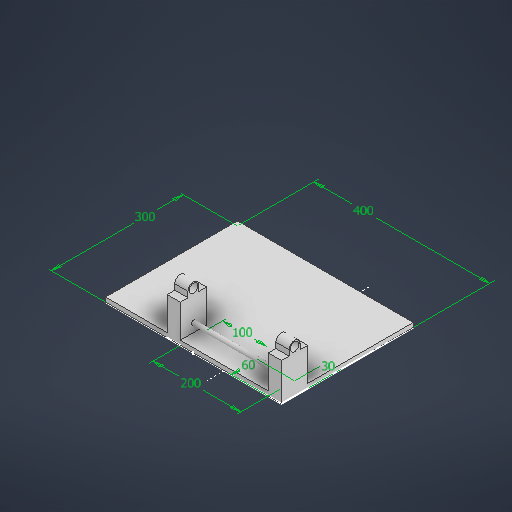
# Autodesk Inventor part: base
Saved by Autodesk Inventor 2026.1 (Build 301233020, 233B)
## iProperties
Created: 2025-12-30
Part Number: base
Material: Generic
Document SubType Name: Modeling
Designer: Austin Ngobeni
Density: 1 g/cm^3
Appearance: Default
Author: Austin Ngobeni
Autodesk Inventor part; units mm, degrees
ref_plane "YZ Plane" through (0, 0, 0) normal (1, 0, 0) x (0, 1, 0)
ref_plane "XZ Plane" through (0, 0, 0) normal (0, 1, 0) x (-1, 0, 0)
ref_plane "XY Plane" through (0, 0, 0) normal (0, 0, 1) x (1, 0, 0)
sketch "Sketch1" plane through (0, 0, 0) normal (0, 1, 0) x (-1, 0, 0)
  line L0 (200, -150) -> (-200, -150)
  line L1 (-200, -150) -> (-200, 150)
  line L2 (-200, 150) -> (200, 150)
  line L3 (200, 150) -> (200, -150)
  line L4 (-200, 150) -> (-170, 150)
  line L5 (-170, 150) -> (-170, 90)
  line L6 (-170, 90) -> (-200, 90)
  line L7 (-200, 90) -> (-200, 150)
  line L8 (60, 150) -> (30, 150)
  line L9 (30, 150) -> (30, 90)
  line L10 (30, 90) -> (60, 90)
  line L11 (60, 90) -> (60, 150)
  line L12 (-70, 187.6664) -> (-70, -178.9653) construction
  point P0 (0, 0)
  point P1 (0, 150)
  point P2 (200, 0)
  point P3 (45, 90)
  point P4 (-185, 90)
  point P5 (-170, 120)
  dimension "d0" = 300
  dimension "d1" = 400
  dimension "d2" = 30
  dimension "d3" = 60
  dimension "d4" = 200
  dimension "d17" = 100
  constraints: 26 end point, 6 parallel, 5 midpoint, 4 perpendicular, 3 horizontal, 2 horizontal alignment, 1 collinear, 1 point on line, 1 vertical alignment
  measures "d0" distance of L2.end L0.start
  measures "d1" distance of L0.start L0.end
  measures "d2" distance of L5.end L6.end
  measures "d3" distance of L4.end L5.end
  measures "d4" distance from line of L9 point (-170, 120)
  measures "d17" distance between parallel lines of L12 L9
extrude "Extrusion1" add sketch "Sketch1" along normal blind 10 contours L0 L1 L6 L5 L2 L9 L10 L11 L3
extrude "Extrusion2" add sketch "Sketch1" along normal blind 80 contours L1 L2 L5 L6 | L11 L10 L9 L2
sketch "Sketch2" plane through (-30, 10, 90) normal (1, 0, 0) x (0, 0, -1)
  circle A0 centre (-30, 20) radius 5
  line L0 (-60, 0) -> (-60, 70) projected
  line L1 (-60, 0) -> (0, 0) projected
  point P0 (90, -10)
  dimension "d9" = 10
  dimension "d10" = 30
  dimension "d11" = 20
  constraints: 1 centre point
  measures "d9" diameter of A0
  measures "d10" distance from line of L0 A0.centre
  measures "d11" distance from line of L1 A0.centre
extrude "Extrusion3" add sketch "Sketch2" along normal up to surface (200 mm away)
sketch "Sketch3" plane through (-60, 10, 150) normal (-1, 0, 0) x (0, 0, 1)
  line L0 (-59.7389, 70) -> (0, 70)
  line L1 (0, 70) -> (0, 75)
  line L2 (-59.7389, 75) -> (-59.7389, 70)
  arc A0 (-17.3694, 87.5) -> (-42.3694, 87.5) centre (-29.8694, 87.5) ccw
  line L3 (-42.3694, 87.5) -> (-42.3694, 75)
  line L4 (-17.3694, 87.5) -> (-17.3694, 75)
  line L5 (0, 75) -> (-17.3694, 75)
  line L6 (-42.3694, 75) -> (-59.7389, 75)
  circle A1 centre (-29.8694, 87.5) radius 10
  point P0 (-150, -10)
  point P1 (-60, 70)
  point P2 (0, 72.5)
  dimension "d14" = 5
  dimension "d15" = 25
  dimension "d16" = 20
  constraints: 14 end point, 4 tangent, 3 parallel, 3 perpendicular, 2 centre point, 2 point on circle, 1 coincident, 1 horizontal, 1 horizontal alignment, 1 midpoint, 1 vertical, 1 vertical alignment
  measures "d14" distance of L2.start L0.start
  measures "d15" diameter of A0
  measures "d16" diameter of A1
extrude "Extrusion4" add sketch "Sketch3" against normal up to surface (30 mm away)
sketch "Sketch4" plane through (200, 0, 150) normal (1, 0, 0) x (0, 0, -1)
  line L0 (0, 80) -> (60, 80) projected
  line L1 (59.7389, 80) -> (59.7389, 85) projected
  line L2 (59.7389, 85) -> (42.3694, 85) projected
  line L3 (17.3694, 85) -> (0, 85) projected
  line L4 (17.3694, 97.5) -> (17.3694, 85) projected
  circle A0 centre (29.8694, 97.5) radius 10 projected
  arc A1 (42.3694, 97.5) -> (17.3694, 97.5) centre (29.8694, 97.5) ccw projected
  line L5 (42.3694, 85) -> (42.3694, 97.5) projected
  line L6 (0, 85) -> (0, 80)
  point P0 (150, 0)
  constraints: 2 end point, 1 perpendicular
extrude "Extrusion5" add sketch "Sketch4" against normal up to surface (30 mm away)
body "Solid1"
